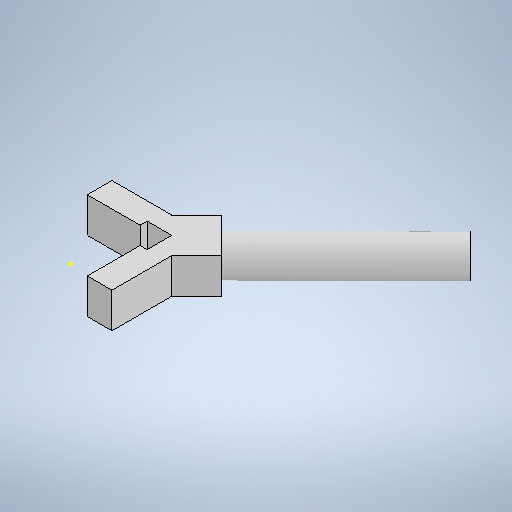
# Autodesk Inventor part: Součást3
Saved by Autodesk Inventor 2025 (Build 290162000, 162)
## iProperties
Created: 2025-05-08
Part Number: Součást3
Material: Všeobecné
Document SubType Name: Modeling
Designer: zdene
Mass: 7.89123 g
Surface Area: 36.6507 cm^2
Volume: 7.89123 cm^3
Density: 1 g/cm^3
Appearance: Výchozí
Author: zdene
Autodesk Inventor part; units mm, degrees
ref_plane "YZ Plane" through (0, 0, 0) normal (1, 0, 0) x (0, 1, 0)
ref_plane "XZ Plane" through (0, 0, 0) normal (0, 1, 0) x (-1, 0, 0)
ref_plane "XY Plane" through (0, 0, 0) normal (0, 0, 1) x (1, 0, 0)
sketch "Náčrt1" plane through (0, 0, 0) normal (0, 0, 1) x (1, 0, 0)
  point P0 (0, 0)
sketch "Náčrt2" plane through (0, 0, 0) normal (0, 0, 1) x (1, 0, 0)
  line L0 (17.2004, -10.497) -> (22.2004, -10.497)
  line L1 (-4.7996, 11.503) -> (-4.7996, 16.503)
  line L2 (-4.7996, 11.503) -> (17.2004, 11.503)
  line L3 (17.2004, -10.497) -> (17.2004, 11.503)
  line L4 (22.2004, -10.497) -> (22.2004, 11.503)
  line L5 (-4.7996, 16.503) -> (22.2004, 16.503)
  line L6 (22.2004, 11.503) -> (22.2004, 16.503)
  point P0 (0, 0)
  point P1 (15.2004, 9.503)
  constraints: 14 end point, 3 perpendicular, 2 horizontal
extrude "Vysunutí1" add sketch "Náčrt2" along normal blind 10
sketch "Náčrt3" plane through (0, 0, 10) normal (0, 0, 1) x (1, 0, 0)
  line L0 (17.2004, 11.503) -> (17.2004, -10.497) projected
  line L1 (22.2004, -10.497) -> (22.2004, 16.503) projected
  line L2 (22.2004, 16.503) -> (-4.7996, 16.503) projected
  line L3 (22.2004, 6.4599) -> (12.2431, 16.503)
  line L4 (12.2431, 16.503) -> (19.3444, 23.5436)
  line L5 (19.3444, 23.5436) -> (29.3017, 13.5006)
  line L6 (29.3017, 13.5006) -> (22.2004, 6.4599)
  point P0 (0, 0)
  constraints: 8 end point, 2 parallel, 2 point on line, 1 perpendicular
extrude "Vysunutí2" add sketch "Náčrt3" against normal blind 10 contours L1 L2 L4 L5 L6
sketch "Náčrt4" plane through (29.3017, 13.5006, 10) normal (0.7101, 0.7041, 0) x (0, 0, -1)
  point P0 (10, 11.0432)
sketch "Náčrt5" plane through (29.3017, 13.5006, 10) normal (0.7101, 0.7041, 0) x (0, 0, -1)
  line L0 (10, 0) -> (0, 0) projected
  line L1 (10, 22.5911) -> (10, 7.1016) projected
  line L2 (0, 14.1425) -> (10, 14.1425) projected
  line L3 (10, 7.1016) -> (10, -8.5213) projected
  line L4 (10, 7.1016) -> (0, 7.1016) projected
  circle A0 centre (5, 7.1016) radius 5
  point P0 (10, 11.0432)
  constraints: 1 centre point, 1 midpoint
extrude "Vysunutí3" add sketch "Náčrt5" along normal blind 50
sketch "Náčrt6" plane through (0, 0, 10) normal (0, 0, 1) x (1, 0, 0)
  line L0 (17.2004, 11.503) -> (17.2004, -10.497) projected
  line L1 (17.2004, -10.497) -> (17.2004, 4.503)
  line L2 (17.2004, 4.503) -> (15.2004, 4.503)
  line L3 (15.2004, 4.503) -> (15.2004, -10.497)
  line L4 (15.2004, -10.497) -> (17.2004, -10.497)
  line L5 (-4.7996, 11.503) -> (17.2004, 11.503) projected
  line L6 (-4.7996, 11.503) -> (-4.7996, 9.503)
  line L7 (-4.7996, 9.503) -> (10.2004, 9.503)
  line L8 (10.2004, 9.503) -> (10.2004, 11.503)
  line L9 (10.2004, 11.503) -> (-4.7996, 11.503)
  point P0 (0, 0)
  constraints: 16 end point, 2 horizontal, 2 perpendicular, 2 point on line, 2 vertical, 1 collinear
extrude "Vysunutí4" add sketch "Náčrt6" against normal blind 10
